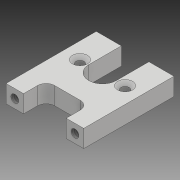
# Autodesk Inventor part: mount_motor_side
Saved by Autodesk Inventor 2017 SP1 (Build 210196100, 196)
## iProperties
Created: 2018-01-19
Part Number: mount_motor_side
Material: Generic
Document SubType Name: Modeling
Designer: Tomasz
Density: 1 g/cm^3
Appearance: Default
Author: Tomasz
Autodesk Inventor part; units mm, degrees
ref_plane "YZ Plane" through (0, 0, 0) normal (1, 0, 0) x (0, 1, 0)
ref_plane "XZ Plane" through (0, 0, 0) normal (0, 1, 0) x (-1, 0, 0)
ref_plane "XY Plane" through (0, 0, 0) normal (0, 0, 1) x (1, 0, 0)
sketch "Sketch1" plane through (0, 0, 0) normal (0, 0, 1) x (1, 0, 0)
  line L0 (15.5, 0) -> (15.5, 18)
  line L1 (0, 18) -> (0, 0)
  line L2 (7.75, 16.4813) -> (7.75, -1.3789) construction
  arc A0 (5, 11.5) -> (10.5, 11.5) centre (7.75, 11.5) ccw
  line L3 (5, 11.5) -> (5, 18)
  line L4 (10.5, 11.5) -> (10.5, 18)
  line L5 (15.5, 18) -> (10.5, 18)
  line L6 (5, 18) -> (0, 18)
  line L7 (3.5, 0) -> (3.5, 2.8)
  line L8 (5.2, 4.5) -> (10.3, 4.5)
  line L9 (12, 2.8) -> (12, 0)
  line L10 (0, 0) -> (3.5, 0)
  line L11 (12, 0) -> (15.5, 0)
  arc A1 (5.2, 4.5) -> (3.5, 2.8) centre (5.2, 2.8) ccw
  arc A2 (12, 2.8) -> (10.3, 4.5) centre (10.3, 2.8) ccw
  line L12 (1.3235, 11.5) -> (14.2571, 11.5) construction
  point P0 (3.25, 11.5)
  point P1 (12.25, 11.5)
  dimension "d0" = 15.5
  dimension "d1" = 18
  dimension "d3" = 5.5
  dimension "d4" = 6.5
  dimension "d5" = 4.5
  dimension "d6" = 8.5
  dimension "d7" = 1.7
  dimension "d8" = 9
  constraints: 26 end point, 9 perpendicular, 6 point on circle, 6 point on line, 6 tangent, 5 parallel, 3 centre point, 3 horizontal, 1 equal radius, 1 symmetric about line, 1 vertical, 3 other
  measures "d0" distance of L1.end L0.start
  measures "d1" distance of L1.start L1.end
  measures "d3" diameter of A0
  measures "d4" distance from line of A0.centre L6
  measures "d5" distance between parallel lines of L10 L8
  measures "d6" distance between parallel lines of L9 L7
  measures "d7" radius of A1
  measures "d8" distance of point (12.25, 11.5) point (3.25, 11.5)
sketch "Sketch2" plane through (0, 0, 0) normal (0, 0, 1) x (1, 0, 0)
  line L0 (0, 18) -> (0, 0) projected
  line L1 (5, 18) -> (0, 18) projected
  line L2 (5, 11.5) -> (5, 18) projected
  arc A0 (5, 11.5) -> (10.5, 11.5) centre (7.75, 11.5) ccw projected
  line L3 (10.5, 11.5) -> (10.5, 18) projected
  line L4 (15.5, 18) -> (10.5, 18) projected
  line L5 (15.5, 0) -> (15.5, 18) projected
  line L6 (12, 2.8) -> (12, 0) projected
  line L7 (12, 0) -> (15.5, 0) projected
  arc A1 (12, 2.8) -> (10.3, 4.5) centre (10.3, 2.8) ccw projected
  line L8 (5.2, 4.5) -> (10.3, 4.5) projected
  arc A2 (5.2, 4.5) -> (3.5, 2.8) centre (5.2, 2.8) ccw projected
  line L9 (3.5, 0) -> (3.5, 2.8) projected
  line L10 (0, 0) -> (3.5, 0) projected
extrude "Extrusion1" add sketch "Sketch2" along normal blind 3.5
sketch "Sketch3" plane through (0, 0, 3.5) normal (0, 0, 1) x (1, 0, 0)
  point P0 (0, 0)
  point P1 (3.25, 11.5)
  point P2 (12.25, 11.5)
hole "Hole1" at (3.25, 11.5, 3.5) at (12.25, 11.5, 3.5) direction (0, 0, -1) diameter 1.6 end through all countersink diameter 3 countersink angle 90
sketch "Sketch4" plane through (0, 18, 0) normal (0, 1, 0) x (1, 0, 0)
  line L0 (0, 0) -> (0, -3.5) projected
  line L1 (0, -1.75) -> (15.5, -1.75) construction
  line L2 (15.5, 0) -> (15.5, -3.5) projected
  line L3 (5.2, -3.5) -> (10.3, -3.5) projected
  line L4 (7.75, -3.5) -> (7.75, 0) construction
  point P0 (2.5, -1.75)
  point P1 (13, -1.75)
  dimension "d18" = 10.5
  constraints: 4 end point, 3 midpoint, 2 point on line, 1 symmetric about line, 1 vertical
  measures "d18" distance of point (13, -1.75) point (2.5, -1.75)
hole "Hole2" at (2.5, 18, 1.75) at (13, 18, 1.75) direction (0, -1, 0) diameter 1.567 depth 4 tip angle 118 thread size "M2x0.4" class "6H" standard "ANSI Metric M Profile"
sketch "Sketch5" plane through (0, 0, 0) normal (0, -1, 0) x (1, 0, 0)
  line L0 (0, 0) -> (0, 3.5) projected
  line L1 (0, 1.75) -> (15.5, 1.75) construction
  line L2 (15.5, 0) -> (15.5, 3.5) projected
  line L3 (5, 3.5) -> (10.5, 3.5) projected
  line L4 (7.75, 3.5) -> (7.75, 0) construction
  line L5 (10.5, 0) -> (5, 0) projected
  point P0 (1.75, 1.75)
  point P1 (13.75, 1.75)
  dimension "d26" = 12
  constraints: 4 end point, 4 midpoint, 2 point on line, 1 symmetric about line
  measures "d26" distance of point (13.75, 1.75) point (1.75, 1.75)
hole "Hole3" at (1.75, 0, 1.75) at (13.75, 0, 1.75) direction (0, 1, 0) diameter 1.567 depth 8 tip angle 118 thread size "M2x0.4" class "6H" standard "ANSI Metric M Profile"
body "Solid1"
